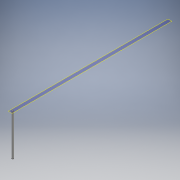
# Autodesk Inventor part: eje codo
Saved by Autodesk Inventor 2016 (Build 200138000, 138)
## iProperties
Created: 2016-08-18
Part Number: eje codo
Material: Generic
Document SubType Name: Modeling
Designer: Admin
Density: 1 g/cm^3
Appearance: Default
Author: Admin
Autodesk Inventor part; units mm, degrees
ref_plane "YZ Plane" through (0, 0, 0) normal (1, 0, 0) x (0, 1, 0)
ref_plane "XZ Plane" through (0, 0, 0) normal (0, 1, 0) x (-1, 0, 0)
ref_plane "XY Plane" through (0, 0, 0) normal (0, 0, 1) x (1, 0, 0)
ref_plane "Work Plane1" through (51.8897, 546.9908, 132) normal (0, 0, -1) x (0.9987207, -0.0505673, 0)
sketch "Sketch1" plane through (51.8897, 546.9908, 132) normal (0, 0, -1) x (0.9987207, -0.0505673, 0)
  circle A0 centre (6, 516) radius 3
  point P0 (-24.1635, 548.9149)
  dimension "d0" = 6
  constraints: 1 centre point
  measures "d0" diameter of A0
extrude "Extrusion1" add sketch "Sketch1" along normal blind 142
body "Solid1"
